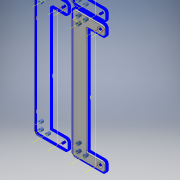
# Autodesk Inventor part: nuc_fix_v2
Saved by Autodesk Inventor 2018 (Build 220112000, 112)
## iProperties
Created: 2018-04-24
Part Number: nuc_fix_v2
Material: Generic
Document SubType Name: Modeling
Designer: medrimonia
Density: 1 g/cm^3
Appearance: Default
Vendor: Rhoban
Mass: 9.23554 g
Surface Area: 59.4529 cm^2
Volume: 9.23554 cm^3
width: 8.900 mm
piano_wire_holes_spacing: 7,500 mm
holes_spacing: 125,000 mm
Author: medrimonia
Autodesk Inventor part; units mm, degrees
ref_plane "YZ Plane" through (0, 0, 0) normal (1, 0, 0) x (0, 1, 0)
ref_plane "XZ Plane" through (0, 0, 0) normal (0, 1, 0) x (-1, 0, 0)
ref_plane "XY Plane" through (0, 0, 0) normal (0, 0, 1) x (1, 0, 0)
sketch "Sketch1" plane through (0, 0, 0) normal (0, 1, 0) x (-1, 0, 0)
  line L0 (0, -62.5) -> (0, 62.5) construction
  line L1 (-4.45, 66.95) -> (-4.45, 58.05)
  line L2 (-4.45, 58.05) -> (14.5, 58.05)
  line L3 (14.5, 58.05) -> (14.5, -58.05)
  line L4 (14.5, -58.05) -> (-4.45, -58.05)
  line L5 (-4.45, -58.05) -> (-4.45, -66.95)
  line L6 (-4.45, -66.95) -> (28.4, -66.95)
  line L7 (28.4, -66.95) -> (28.4, 66.95)
  line L8 (28.4, 66.95) -> (-4.45, 66.95)
  line L9 (0, 62.5) -> (-4.45, 62.5) construction
  line L10 (-4.45, -62.5) -> (0, -62.5) construction
  point P0 (0, 0)
  point P1 (0, 0)
  dimension "d0" = 125
  dimension "d1" = 4.45
  dimension "d2" = 4.45
  dimension "d3" = 13.9
  dimension "d4" = 14.5
  dimension "d5" = 4.45
  constraints: 22 end point, 4 perpendicular, 3 coincident, 3 horizontal, 3 midpoint, 3 vertical, 2 parallel
  measures "d0" distance of L0.start L0.end
  measures "d1" distance of L0.end L9.end
  measures "d2" distance between parallel lines of L9 L2
  measures "d3" distance between parallel lines of L7 L3
  measures "d4" distance between parallel lines of L3 L0
  measures "d5" distance between parallel lines of L10 L4
extrude "Extrusion1" add sketch "Sketch1" along normal blind 3
hole "Hole1" at (0, 0, 62.5) at (0, 0, -62.5) direction (0, 1, 0) diameter 5 end through all
fillet "Fillet1" radius 1.5 8 edges at (-14.5, 1.5, 58.05) (-28.4, 1.5, 66.95) (-14.5, 1.5, -58.05) (-28.4, 1.5, -66.95) (4.45, 1.5, -58.05) (4.45, 1.5, -66.95) (4.45, 1.5, 58.05) (4.45, 1.5, 66.95)
sketch "Sketch2" plane through (0, 3, 0) normal (0, 1, 0) x (1, 0, 0)
  arc A0 (-26.9, 66.95) -> (-28.4, 65.45) centre (-26.9, 65.45) ccw projected
  line L0 (-28.4, 65.45) -> (-28.4, -65.45) projected
  arc A1 (-28.4, -65.45) -> (-26.9, -66.95) centre (-26.9, -65.45) ccw projected
  line L1 (-26.9, -66.95) -> (2.95, -66.95) projected
  line L2 (4.45, -65.45) -> (4.45, -59.55) projected
  line L3 (2.95, -58.05) -> (-13, -58.05) projected
  arc A2 (-14.5, -56.55) -> (-13, -58.05) centre (-13, -56.55) ccw projected
  line L4 (-14.5, -56.55) -> (-14.5, 56.55) projected
  arc A3 (-13, 58.05) -> (-14.5, 56.55) centre (-13, 56.55) ccw projected
  line L5 (-13, 58.05) -> (2.95, 58.05) projected
  line L6 (4.45, 59.55) -> (4.45, 65.45) projected
  line L7 (2.95, 66.95) -> (-26.9, 66.95) projected
  circle A4 centre (0, -62.5) radius 2.5 projected
  circle A5 centre (0, 62.5) radius 2.5 projected
  line L8 (4.45, -65.45) -> (4.45, -59.55) construction
  line L9 (4.45, -62.5) -> (-28.4, -62.5) construction
  line L10 (-28.4, 65.45) -> (-28.4, -65.45) construction
  line L11 (4.45, 59.55) -> (4.45, 65.45) construction
  line L12 (4.45, 62.5) -> (-28.4, 62.5) construction
  line L13 (-14.5, 0) -> (-28.4, 0) construction
  line L14 (2.95, 66.95) -> (-26.9, 66.95) construction
  line L15 (-26.9, -66.95) -> (2.95, -66.95) construction
  line L16 (-23.95, 66.95) -> (-23.95, -66.95) construction
  arc A6 (2.95, -66.95) -> (4.45, -65.45) centre (2.95, -65.45) ccw projected
  arc A7 (4.45, -59.55) -> (2.95, -58.05) centre (2.95, -59.55) ccw projected
  arc A8 (2.95, 58.05) -> (4.45, 59.55) centre (2.95, 59.55) ccw projected
  arc A9 (4.45, 65.45) -> (2.95, 66.95) centre (2.95, 65.45) ccw projected
  point P0 (0, 0)
  point P1 (4.45, -66.95)
  point P2 (4.45, -58.05)
  point P3 (4.45, 58.05)
  point P4 (4.45, 66.95)
  point P5 (-21.45, 0)
  point P6 (-23.95, -62.5)
  point P7 (-16.45, -62.5)
  point P8 (-23.95, -55)
  point P9 (-23.95, 62.5)
  point P10 (-16.45, 62.5)
  point P11 (-23.95, 55)
  dimension "d7" = 0
  dimension "d17" = 7.5
  dimension "d25" = 4.45
  dimension "d26" = 7.5
  constraints: 8 end point, 8 point on line, 5 midpoint, 3 symmetric about line, 1 horizontal, 1 perpendicular, 1 vertical
  measures "d17" distance of point (-23.95, -62.5) point (-23.95, -55)
  measures "d25" distance between parallel lines of L10 L16
  measures "d26" distance from line of point (-16.45, -62.5) L16
hole "Hole2" at (-23.95, 3, 62.5) at (-16.45, 3, 62.5) at (-23.95, 3, 55) at (-23.95, 3, -55) at (-23.95, 3, -62.5) at (-16.45, 3, -62.5) direction (0, -1, 0) diameter 3 end through all
equation "\"d0\" = holes_spacing"
equation "\"d1\" = 0.5 * width"
equation "\"d2\" = 0.5 * width"
equation "\"d3\" = width + back_extra_width"
equation "\"d4\" = holes_2_back"
equation "\"d5\" = 0.5 * width"
equation "\"d6\" = thickness"
equation "\"d17\" = piano_wire_holes_spacing"
equation "\"d25\" = 0.5 * width"
equation "\"d26\" = piano_wire_holes_spacing"
equation "\"thickness\" = 3"
equation "\"holes_spacing\" = 125"
equation "\"holes_2_back\" = 14.5"
equation "\"width\" = 8.9"
equation "\"piano_wire_holes_spacing\" = 7.5"
equation "\"back_extra_width\" = 5"
body "Solid1"
